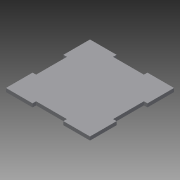
# Autodesk Inventor part: outside_box_top_bot
Saved by Autodesk Inventor 2013 (Build 170138000, 138)
## iProperties
Created: 2014-05-23
Part Number: outside_box_top_bot
Material: Generic
Document SubType Name: Modeling
Designer: balogh
Density: 1 g/cm^3
Author: balogh
Autodesk Inventor part; units mm, degrees
ref_plane "YZ Plane" through (0, 0, 0) normal (1, 0, 0) x (0, 1, 0)
ref_plane "XZ Plane" through (0, 0, 0) normal (0, 1, 0) x (-1, 0, 0)
ref_plane "XY Plane" through (0, 0, 0) normal (0, 0, 1) x (1, 0, 0)
sketch "Sketch1" plane through (0, 0, 0) normal (0, 0, 1) x (1, 0, 0)
  line L0 (12.7, -31.75) -> (12.7, -34.6456)
  line L1 (12.7, -34.6456) -> (34.6456, -34.6456)
  line L2 (34.6456, -34.6456) -> (34.6456, -12.7)
  line L3 (34.6456, -12.7) -> (31.75, -12.7)
  line L4 (31.75, -12.7) -> (31.75, 12.7)
  line L5 (31.75, 12.7) -> (34.6456, 12.7)
  line L6 (34.6456, 12.7) -> (34.6456, 34.6456)
  line L7 (34.6456, 34.6456) -> (12.7, 34.6456)
  line L8 (12.7, 34.6456) -> (12.7, 31.75)
  line L9 (12.7, 31.75) -> (-12.7, 31.75)
  line L10 (-12.7, 31.75) -> (-12.7, 34.6456)
  line L11 (-12.7, 34.6456) -> (-34.6456, 34.6456)
  line L12 (-34.6456, 34.6456) -> (-34.6456, 12.7)
  line L13 (-34.6456, 12.7) -> (-31.75, 12.7)
  line L14 (-31.75, 12.7) -> (-31.75, -12.7)
  line L15 (-31.75, -12.7) -> (-34.6456, -12.7)
  line L16 (-34.6456, -12.7) -> (-34.6456, -34.6456)
  line L17 (-34.6456, -34.6456) -> (-12.7, -34.6456)
  line L18 (-12.7, -34.6456) -> (-12.7, -31.75)
  line L19 (-12.7, -31.75) -> (12.7, -31.75)
  point P0 (0, 0)
  constraints: 40 end point, 11 parallel, 6 perpendicular, 2 collinear
extrude "Extrusion1" add sketch "Sketch1" along normal blind 2.8956
body "Solid1"
